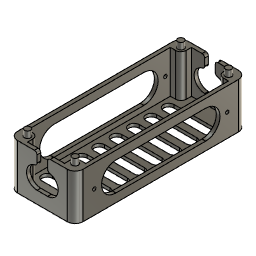
monitor-power-tower v7 (Autodesk Fusion 360 design; units mm, degrees)
Autodesk Fusion 360 part; units mm, degrees
note: some values were not read from the file. Set by a fixed rule: which sketch regions a step uses.
sketch "top" plane through (0, 0, 0) normal (0, 0, 1) x (1, 0, 0)
  line L0 (-27.5, 77.5) -> (27.5, 77.5)
  line L1 (27.5, 77.5) -> (27.5, -77.5)
  line L2 (27.5, -77.5) -> (-27.5, -77.5)
  line L3 (-27.5, -77.5) -> (-27.5, 77.5)
  line L4 (31, -81) -> (-31, -81)
  line L5 (-31, -81) -> (-31, 81)
  line L6 (-31, 81) -> (31, 81)
  line L7 (31, 81) -> (31, -81)
  line L8 (0, 77.5) -> (0, -77.5) construction
  line L9 (-27.5, 0) -> (27.5, 0) construction
  circle A0 centre (22.5, 72.5) radius 1.55
  circle A1 centre (22.5, 72.5) radius 3
  circle A2 centre (22.5, 72.5) radius 5
  circle A3 centre (-22.5, 72.5) radius 5
  circle A4 centre (-22.5, 72.5) radius 3
  circle A5 centre (-22.5, 72.5) radius 1.55
  circle A6 centre (-22.5, -72.5) radius 5
  circle A7 centre (-22.5, -72.5) radius 3
  circle A8 centre (-22.5, -72.5) radius 1.55
  circle A9 centre (22.5, -72.5) radius 5
  circle A10 centre (22.5, -72.5) radius 3
  circle A11 centre (22.5, -72.5) radius 1.55
  line L10 (22.5, 72.5) -> (22.5, 67.5)
  line L11 (22.5, 72.5) -> (17.5, 72.5)
  line L12 (22.5, 67.5) -> (27.5, 67.5)
  line L13 (17.5, 72.5) -> (17.5, 77.5)
  line L14 (-17.5, 72.5) -> (-17.5, 77.5)
  line L15 (-22.5, 67.5) -> (-27.5, 67.5)
  line L16 (22.5, -67.5) -> (27.5, -67.5)
  line L17 (17.5, -72.5) -> (17.5, -77.5)
  line L18 (-17.5, -72.5) -> (-17.5, -77.5)
  line L19 (-22.5, -67.5) -> (-27.5, -67.5)
  line L20 (-19, 52.5) -> (19, 52.5)
  arc A12 (19, 52.5) -> (19, 62.5) centre (19, 57.5) ccw
  line L21 (19, 62.5) -> (-19, 62.5)
  arc A13 (-19, 62.5) -> (-19, 52.5) centre (-19, 57.5) ccw
  line L22 (-19, 57.5) -> (19, 57.5) construction
  line L23 (0, 62.5) -> (0, 52.5)
  arc A14 (-19, 46.0714) -> (-19, 36.0714) centre (-19, 41.0714) ccw
  line L24 (19, 46.0714) -> (-19, 46.0714)
  line L25 (-19, 36.0714) -> (19, 36.0714)
  arc A15 (19, 36.0714) -> (19, 46.0714) centre (19, 41.0714) ccw
  arc A16 (-19, 29.6429) -> (-19, 19.6429) centre (-19, 24.6429) ccw
  line L26 (19, 29.6429) -> (-19, 29.6429)
  line L27 (-19, 19.6429) -> (19, 19.6429)
  arc A17 (19, 19.6429) -> (19, 29.6429) centre (19, 24.6429) ccw
  arc A18 (-19, 13.2143) -> (-19, 3.2143) centre (-19, 8.2143) ccw
  line L28 (19, 13.2143) -> (-19, 13.2143)
  line L29 (-19, 3.2143) -> (19, 3.2143)
  arc A19 (19, 3.2143) -> (19, 13.2143) centre (19, 8.2143) ccw
  arc A20 (-19, -3.2143) -> (-19, -13.2143) centre (-19, -8.2143) ccw
  line L30 (19, -3.2143) -> (-19, -3.2143)
  line L31 (-19, -13.2143) -> (19, -13.2143)
  arc A21 (19, -13.2143) -> (19, -3.2143) centre (19, -8.2143) ccw
  arc A22 (-19, -19.6429) -> (-19, -29.6429) centre (-19, -24.6429) ccw
  line L32 (19, -19.6429) -> (-19, -19.6429)
  line L33 (-19, -29.6429) -> (19, -29.6429)
  arc A23 (19, -29.6429) -> (19, -19.6429) centre (19, -24.6429) ccw
  arc A24 (-19, -36.0714) -> (-19, -46.0714) centre (-19, -41.0714) ccw
  line L34 (19, -36.0714) -> (-19, -36.0714)
  line L35 (-19, -46.0714) -> (19, -46.0714)
  arc A25 (19, -46.0714) -> (19, -36.0714) centre (19, -41.0714) ccw
  arc A26 (-19, -52.5) -> (-19, -62.5) centre (-19, -57.5) ccw
  line L36 (19, -52.5) -> (-19, -52.5)
  line L37 (-19, -62.5) -> (19, -62.5)
  arc A27 (19, -62.5) -> (19, -52.5) centre (19, -57.5) ccw
  dimension "d1" = 55
  dimension "d2" = 155
  dimension "d3" = -3.5
  dimension "d4" = 3.1
  dimension "d5" = 6
  dimension "d6" = 2
  dimension "d20" = 10
  dimension "d21" = 5
  dimension "d22" = 38
  dimension "d25" = 0
  dimension "d26" = -115
  constraint horizontal L0
  constraint vertical L1
  constraint horizontal L2
  constraint vertical L3
  constraint midpoint L0 L8.start
  constraint midpoint L2 L8.end
  constraint midpoint L3 L9.start
  constraint midpoint L1 L9.end
  constraint concentric A0 A1
  constraint tangent L0 A2
  constraint tangent L1 A2
  constraint midpoint L9 origin
  constraint symmetric L8 A0 A5
  constraint symmetric L8 A1 A4
  constraint symmetric L8 A2 A3
  constraint symmetric L9 A0 A11
  constraint symmetric L9 A1 A10
  constraint symmetric L9 A2 A9
  constraint symmetric L9 A3 A6
  constraint symmetric L9 A4 A7
  constraint symmetric L9 A5 A8
  constraint coincident A0.centre A1.centre
  constraint coincident A2 L10.end
  constraint vertical L10
  constraint coincident A2 L11.end
  constraint perpendicular L10 L11
  constraint coincident L1 L12.end
  constraint tangent A2 L12
  constraint coincident L0 L13.end
  constraint tangent A2 L13
  constraint symmetric L8 L10.end L15.start
  constraint symmetric L8 L11.end L14.start
  constraint symmetric L8 L12.end L15.end
  constraint symmetric L8 L13.end L14.end
  constraint symmetric L9 L10.end L16.start
  constraint symmetric L9 L11.end L17.start
  constraint symmetric L9 L12.end L16.end
  constraint symmetric L9 L13.end L17.end
  constraint symmetric L9 L14.start L18.start
  constraint symmetric L9 L14.end L18.end
  constraint symmetric L9 L15.start L19.start
  constraint symmetric L9 L15.end L19.end
  constraint tangent L20 A12
  constraint tangent A12 L21
  constraint parallel L20 L21
  constraint tangent L21 A13
  constraint tangent L20 A13
  constraint perpendicular L3 L22
  constraint midpoint L21 L23.start
  constraint midpoint L20 L23.end
  constraint coincident L8 L23.start
  measures "d1" distance of L0.start L0.end
  measures "d2" distance of L0.end L1.end
  measures "d4" diameter of A0
  measures "d5" diameter of A1
  measures "d20" diameter of A12
  measures "d21" distance of L15 L21
  measures "d22" distance of A13.centre A12.centre
extrude "Extrude1" add sketch "top" along normal blind 3 contours L0 A3 L14 | L0 L1 L2 L3 A2 A3 A6 A9 L12 L13 L14 L15 L16 L17 L18 L19 | L0 A2 L13 | L0 L3 A3 | A3 | L0 L1 A2 | A1 A2 L10 L11 | A1 A2 L10 L11 | L3 A3 L15 | L1 A2 L12 | A0 A1 L10 L11 | A0 A1 L10 L11 | A0 L10 L11 | A0 L10 L11 | L3 A6 L19 | L1 A9 L16 | L2 L3 A6 | A6 | A9 | L1 L2 A9 | L2 A6 L18 | L2 A9 L17 | L4 L5 L6 L7 | A4 | A5 | A7 | A8 | A10 | A11 | L20 L21 A13 L23 | L20 A12 L21 L23 | A14 L24 L25 A15 | A16 L26 L27 A17 | A18 L28 L29 A19 | A20 L30 L31 A21 | A22 L32 L33 A23 | A24 L34 L35 A25 | A26 L36 L37 A27
extrude "Extrude2" add sketch "top" along normal blind 40 from surface at 3 contours L4 L5 L6 L7
extrude "Extrude3" add sketch "top" along normal up to surface (43 mm away) contours L0 A3 L14 | L0 A2 L13 | L0 L3 A3 | A3 | L0 L1 A2 | A1 A2 L10 L11 | A1 A2 L10 L11 | L3 A3 L15 | L1 A2 L12 | A0 A1 L10 L11 | A0 A1 L10 L11 | A0 L10 L11 | A0 L10 L11 | L3 A6 L19 | L1 A9 L16 | L2 L3 A6 | A6 | A9 | L1 L2 A9 | L2 A6 L18 | L2 A9 L17 | A4 | A5 | A7 | A8 | A10 | A11
extrude "Extrude4" cut sketch "top" against normal blind 15 from surface at 43 contours A0 L10 L11 | A0 L10 L11 | A5 | A8 | A11
extrude "Extrude5" cut sketch "top" against normal blind 2 from surface at 43 contours A0 A1 L10 L11 | A0 A1 L10 L11 | A4 | A7 | A10
extrude "Extrude6" cut sketch "top" along normal up to surface (3 mm away) contours L20 L21 A13 L23 | L20 A12 L21 L23 | A14 L24 L25 A15 | A16 L26 L27 A17 | A18 L28 L29 A19 | A20 L30 L31 A21 | A22 L32 L33 A23 | A24 L34 L35 A25 | A26 L36 L37 A27
sketch "front" plane through (0, -81, 0) normal (0, -1, 0) x (1, 0, 0)
  line L0 (-31, 0) -> (31, 0)
  line L1 (31, 0) -> (31, 43)
  line L2 (31, 43) -> (-31, 43)
  line L3 (-31, 43) -> (-31, 0)
  line L4 (-31, 43) -> (31, 43)
  line L5 (-31, 0) -> (-31, 43)
  line L6 (31, 0) -> (-31, 0)
  line L7 (31, 0) -> (31, 43)
  line L8 (0, 43) -> (0, 0) construction
  line L9 (-31, 21.5) -> (31, 21.5) construction
  line L10 (-5, 11.5) -> (5, 11.5)
  arc A0 (5, 11.5) -> (5, 31.5) centre (5, 21.5) ccw
  line L11 (5, 31.5) -> (-5, 31.5)
  arc A1 (-5, 31.5) -> (-5, 11.5) centre (-5, 21.5) ccw
  line L12 (-5, 21.5) -> (5, 21.5) construction
  line L13 (0, 31.5) -> (0, 11.5) construction
  line L14 (17.5, 3) -> (17.5, 43)
  line L15 (-17.5, 43) -> (-17.5, 3)
  line L16 (-5, 31.5) -> (-5, 43)
  line L17 (5, 31.5) -> (5, 43)
  dimension "d29" = 20
  dimension "d30" = 10
  constraint midpoint L4 L8.start
  constraint coincident L8.end origin
  constraint midpoint L5 L9.start
  constraint midpoint L7 L9.end
  constraint tangent L10 A0
  constraint tangent A0 L11
  constraint parallel L10 L11
  constraint tangent L11 A1
  constraint tangent L10 A1
  constraint coincident L9 A0.centre
  constraint parallel L9 L12
  constraint midpoint L11 L13.start
  constraint midpoint L10 L13.end
  constraint collinear L8 L13
  constraint coincident L4 L16.end
  constraint perpendicular L4 L16
  constraint symmetric L8 L11.end A0.end
  constraint symmetric L8 L16.end L17.end
  measures "d29" diameter of A0
  measures "d30" distance of A1.centre A0.centre
sketch "side" plane through (31, 0, 0) normal (1, 0, 0) x (0, 1, 0)
  line L0 (-81, 0) -> (81, 0)
  line L1 (81, 0) -> (81, 43)
  line L2 (81, 43) -> (-81, 43)
  line L3 (-81, 43) -> (-81, 0)
  line L4 (-81, 43) -> (81, 43)
  line L5 (-81, 0) -> (-81, 43)
  line L6 (81, 0) -> (-81, 0)
  line L7 (81, 0) -> (81, 43)
  line L8 (0, 43) -> (0, 0) construction
  line L9 (-81, 21.5) -> (81, 21.5) construction
  line L10 (-42.5, 8) -> (42.5, 8)
  arc A0 (42.5, 8) -> (42.5, 35) centre (42.5, 21.5) ccw
  line L11 (42.5, 35) -> (-42.5, 35)
  arc A1 (-42.5, 35) -> (-42.5, 8) centre (-42.5, 21.5) ccw
  line L12 (-42.5, 21.5) -> (42.5, 21.5) construction
  circle A2 centre (-62.875, 21.5) radius 1.625
  line L13 (-67.5, 43) -> (-67.5, 3)
  circle A3 centre (62.875, 21.5) radius 1.625
  dimension "d37" = 8
  dimension "d38" = 25
  dimension "d39" = 25
  dimension "d44" = 3.25
  dimension "d45" = 3
  constraint midpoint L4 L8.start
  constraint coincident L8.end origin
  constraint midpoint L5 L9.start
  constraint midpoint L7 L9.end
  constraint tangent L10 A0
  constraint tangent A0 L11
  constraint parallel L10 L11
  constraint tangent L11 A1
  constraint tangent L10 A1
  constraint coincident L9 A0.centre
  constraint parallel L9 L12
  constraint coincident L9 A2.centre
  constraint symmetric L8 A2 A3
  measures "d37" distance of L4 L11
  measures "d38" distance of L7 A0
  measures "d39" distance of L3 A1
  measures "d44" diameter of A2
  measures "d45" distance of A2 L13
extrude "Extrude9" cut sketch "side" against normal up to surface (62 mm away) contours L10 A0 L11 A1
extrude "Extrude10" cut sketch "top" along normal blind 10 contours A0 A1 L10 L11 | A0 A1 L10 L11 | A0 L10 L11 | A0 L10 L11 | A4 | A5 | A7 | A8 | A10 | A11
extrude "Extrude11" cut sketch "side" against normal up to surface (62 mm away) contours A2 | A3
sketch "top-2" plane through (0, 0, 0) normal (0, 0, 1) x (1, 0, 0)
  circle A0 centre (-22.5, 72.5) radius 3
  circle A1 centre (-22.5, 72.5) radius 1.55
  circle A2 centre (-22.5, -72.5) radius 3
  circle A3 centre (-22.5, -72.5) radius 1.55
  circle A4 centre (22.5, -72.5) radius 1.55
  circle A5 centre (22.5, -72.5) radius 3
  circle A6 centre (22.5, 72.5) radius 3
  circle A7 centre (22.5, 72.5) radius 1.55
  line L0 (31, -81) -> (31, 81)
  line L1 (31, 81) -> (-31, 81)
  line L2 (31, 81) -> (-31, 81)
  line L3 (-31, 81) -> (-31, -81)
  line L4 (-27.5, -67.5) -> (-27.5, 67.5)
  line L5 (-31, -81) -> (31, -81)
  line L6 (-31, -81) -> (31, -81)
  line L7 (17.5, -77.5) -> (17.5, -72.5)
  arc A8 (22.5, -67.5) -> (17.5, -72.5) centre (22.5, -72.5) ccw
  line L8 (22.5, -67.5) -> (27.5, -67.5)
  line L9 (27.5, 67.5) -> (27.5, -67.5)
  line L10 (-17.5, -72.5) -> (-17.5, -77.5)
  arc A9 (-17.5, -72.5) -> (-22.5, -67.5) centre (-22.5, -72.5) ccw
  line L11 (-27.5, -67.5) -> (-22.5, -67.5)
  line L12 (-22.5, 67.5) -> (-27.5, 67.5)
  arc A10 (-22.5, 67.5) -> (-17.5, 72.5) centre (-22.5, 72.5) ccw
  line L13 (-17.5, 77.5) -> (-17.5, 72.5)
  line L14 (17.5, 72.5) -> (17.5, 77.5)
  arc A11 (17.5, 72.5) -> (22.5, 67.5) centre (22.5, 72.5) ccw
  line L15 (27.5, 67.5) -> (22.5, 67.5)
  circle A12 centre (22.5, 72.5) radius 2.875
  line L16 (27.5, 0) -> (-27.5, 0) construction
  line L17 (17.5, 72.5) -> (-17.5, 72.5)
  line L18 (17.5, -72.5) -> (-17.5, -72.5)
  line L19 (0, 72.5) -> (0, -72.5) construction
  circle A13 centre (22.5, -72.5) radius 2.875
  circle A14 centre (-22.5, 72.5) radius 2.875
  circle A15 centre (-22.5, -72.5) radius 2.875
  dimension "d48" = 5.75
  constraint concentric A7 A12
  constraint midpoint L9 L16.start
  constraint midpoint L4 L16.end
  constraint coincident L14.start A11.start
  constraint coincident A10.end L13.end
  constraint coincident L7.end A8.end
  constraint coincident L10.start A9.start
  constraint midpoint L17 L19.start
  constraint midpoint L18 L19.end
  constraint symmetric A12 L16 A13
  constraint symmetric A12 L19 A14
  constraint symmetric L19 A13 A15
  measures "d48" diameter of A12
extrude "Extrude12" add sketch "top-2" along normal blind 8 from surface at 41 contours A1 | A3 | A4 | A7 | A12 | A13 | A14 | A15
fillet "Fillet1" radius 7.5 4 edges at (-31, 81, 21.5) (31, 81, 21.5) (31, -81, 21.5) (-31, -81, 21.5)
extrude "Extrude13" cut sketch "front" against normal up to surface (162 mm away) contours L2 L4 L11 L16 L17 | L10 A0 L11 A1
fillet "Fillet4" radius 2.5 8 edges at (-5, -79.25, 43) (5, -79.25, 43) (5, -79.25, 31.5) (-5, -79.25, 31.5) (-5, 79.25, 43) (-5, 79.25, 31.5) (5, 79.25, 43) (5, 79.25, 31.5)
sketch "Sketch6" plane through (0, 0, 0) normal (0, 0, -1) x (1, 0, 0)
  arc A0 (-23.5, 81) -> (-31, 73.5) centre (-23.5, 73.5) ccw
  line L0 (-31, 73.5) -> (-31, -73.5)
  arc A1 (-31, -73.5) -> (-23.5, -81) centre (-23.5, -73.5) ccw
  line L1 (-23.5, -81) -> (23.5, -81)
  arc A2 (23.5, -81) -> (31, -73.5) centre (23.5, -73.5) ccw
  line L2 (31, -73.5) -> (31, 73.5)
  arc A3 (31, 73.5) -> (23.5, 81) centre (23.5, 73.5) ccw
  line L3 (23.5, 81) -> (-23.5, 81)
  circle A4 centre (22.5, 72.5) radius 3
  circle A5 centre (22.5, -72.5) radius 3
  circle A6 centre (-22.5, 72.5) radius 3
  circle A7 centre (-22.5, -72.5) radius 3
  line L4 (19, 19.6429) -> (-19, 19.6429)
  arc A8 (-19, 29.6429) -> (-19, 19.6429) centre (-19, 24.6429) ccw
  line L5 (-19, 29.6429) -> (19, 29.6429)
  arc A9 (19, 19.6429) -> (19, 29.6429) centre (19, 24.6429) ccw
  line L6 (19, -46.0714) -> (-19, -46.0714)
  arc A10 (-19, -36.0714) -> (-19, -46.0714) centre (-19, -41.0714) ccw
  line L7 (-19, -36.0714) -> (19, -36.0714)
  arc A11 (19, -46.0714) -> (19, -36.0714) centre (19, -41.0714) ccw
  line L8 (19, -29.6429) -> (-19, -29.6429)
  arc A12 (-19, -19.6429) -> (-19, -29.6429) centre (-19, -24.6429) ccw
  line L9 (-19, -19.6429) -> (19, -19.6429)
  arc A13 (19, -29.6429) -> (19, -19.6429) centre (19, -24.6429) ccw
  line L10 (19, 36.0714) -> (-19, 36.0714)
  arc A14 (-19, 46.0714) -> (-19, 36.0714) centre (-19, 41.0714) ccw
  line L11 (-19, 46.0714) -> (19, 46.0714)
  arc A15 (19, 36.0714) -> (19, 46.0714) centre (19, 41.0714) ccw
  line L12 (19, 3.2143) -> (-19, 3.2143)
  arc A16 (-19, 13.2143) -> (-19, 3.2143) centre (-19, 8.2143) ccw
  line L13 (-19, 13.2143) -> (19, 13.2143)
  arc A17 (19, 3.2143) -> (19, 13.2143) centre (19, 8.2143) ccw
  line L14 (-19, -52.5) -> (19, -52.5)
  arc A18 (19, -62.5) -> (19, -52.5) centre (19, -57.5) ccw
  line L15 (19, -62.5) -> (-19, -62.5)
  arc A19 (-19, -52.5) -> (-19, -62.5) centre (-19, -57.5) ccw
  line L16 (19, -13.2143) -> (-19, -13.2143)
  arc A20 (-19, -3.2143) -> (-19, -13.2143) centre (-19, -8.2143) ccw
  line L17 (-19, -3.2143) -> (19, -3.2143)
  arc A21 (19, -13.2143) -> (19, -3.2143) centre (19, -8.2143) ccw
  line L18 (19, 52.5) -> (-19, 52.5)
  arc A22 (-19, 62.5) -> (-19, 52.5) centre (-19, 57.5) ccw
  line L19 (-19, 62.5) -> (19, 62.5)
  arc A23 (19, 52.5) -> (19, 62.5) centre (19, 57.5) ccw
  circle A24 centre (-22.5, 72.5) radius 3
  line L20 (23.5, 81) -> (-23.5, 81)
  line L21 (-31, 73.5) -> (-31, -73.5)
  line L22 (31, -73.5) -> (31, 73.5)
  arc A25 (-23.5, 81) -> (-31, 73.5) centre (-23.5, 73.5) ccw
  arc A26 (31, 73.5) -> (23.5, 81) centre (23.5, 73.5) ccw
  arc A27 (23.5, -81) -> (31, -73.5) centre (23.5, -73.5) ccw
  line L23 (-23.5, -81) -> (23.5, -81)
  arc A28 (-31, -73.5) -> (-23.5, -81) centre (-23.5, -73.5) ccw
  line L24 (-31, 0) -> (31, 0) construction
  line L25 (0, 81) -> (0, -81) construction
  circle A29 centre (-22.5, 72.5) radius 3.8
  circle A30 centre (22.5, 72.5) radius 3.8
  circle A31 centre (-22.5, -72.5) radius 3.8
  circle A32 centre (22.5, -72.5) radius 3.8
  dimension "d62" = 0.8
  constraint midpoint L21 L24.start
  constraint midpoint L22 L24.end
  constraint midpoint L20 L25.start
  constraint midpoint L23 L25.end
  constraint symmetric L25 A29 A30
  constraint symmetric L24 A29 A31
  constraint symmetric L24 A30 A32
extrude "Extrude14" cut sketch "Sketch6" against normal up to surface (10 mm away) contours A29 | A30 | A31 | A32
named bodies: "brick-shell"
